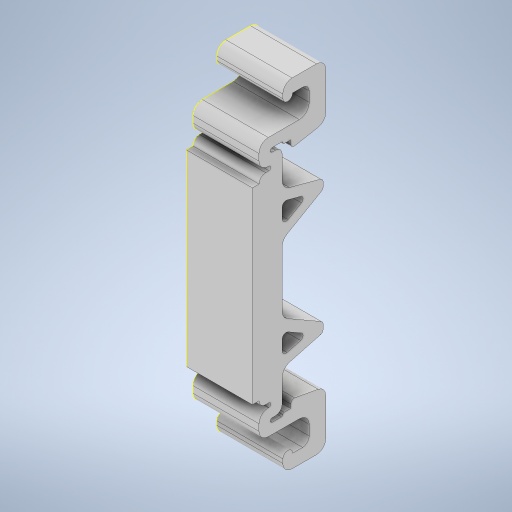
# Autodesk Inventor part: DIN-rail-mount
Saved by Autodesk Inventor 2023 (Build 270158030, 158C)
## iProperties
Created: 2024-03-20
Part Number: DIN-rail-mount
Material: Generic
Document SubType Name: Modeling
Designer: Imogen Heard
Density: 1 g/cm^3
Appearance: Default
Author: Imogen Heard
Autodesk Inventor part; units mm, degrees
ref_plane "YZ Plane" through (0, 0, 0) normal (1, 0, 0) x (0, 1, 0)
ref_plane "XZ Plane" through (0, 0, 0) normal (0, 1, 0) x (-1, 0, 0)
ref_plane "XY Plane" through (0, 0, 0) normal (0, 0, 1) x (1, 0, 0)
sketch "DIN-rail-clip-generic-V1.0" plane through (0, 0, 0) normal (0, 0, 1) x (1, 0, 0)
  line L0 (0, 40.9467) -> (3, 40.9467)
  line L1 (3, 40.9467) -> (3, 17.5)
  line L2 (3, 17.5) -> (0, 17.5)
  line L3 (0, 17.5) -> (0, 40.9467)
  line L4 (0, 35.1) -> (-0.3528, 35.269) construction
  line L5 (-0.3528, 35.269) -> (-1.1784, 35.269) construction
  line L6 (-1.1784, 35.269) -> (-1.277, 34.6657) construction
  line L7 (-1.277, 34.6657) -> (-0.9372, 34.5565) construction
  line L8 (-0.9372, 34.5565) -> (-2.5363, 34.2808) construction
  line L9 (-2.5363, 34.2808) -> (-3.3649, 34.5884) construction
  line L10 (-3.3649, 34.5884) -> (-4.7205, 35.8697) construction
  line L11 (-4.7205, 35.8697) -> (-5.1321, 37.4532) construction
  line L12 (-5.1321, 37.4532) -> (-5.1209, 40.8876) construction
  line L13 (-5.1209, 40.8876) -> (-4.7, 42.1113) construction
  line L14 (-4.7, 42.1113) -> (-3.9, 43.3113) construction
  line L15 (-3.9, 43.3113) -> (-2.1, 44.1113) construction
  line L16 (-2.1, 44.1113) -> (0, 43.5467) construction
  line L17 (0, 43.5467) -> (0.1036, 42.9467) construction
  line L18 (0.1036, 42.9467) -> (-0.2, 41.9467) construction
  line L19 (-0.2, 41.9467) -> (-1.1, 42.4004) construction
  line L20 (-1.1, 42.4004) -> (-2.3, 42.4379) construction
  spline S0 degree 4 poles (0, 35.1) (-0.3528, 35.269) (-1.1784, 35.269) (-1.277, 34.6657) (-0.9372, 34.5565) (-2.5363, 34.2808) (-3.3649, 34.5884) (-4.7205, 35.8697) (-5.1321, 37.4532) (-5.1209, 40.8876) (-4.7, 42.1113) (-3.9, 43.3113) (-2.1, 44.1113) (0, 43.5467) (0.1036, 42.9467) (-0.2, 41.9467) (-1.1, 42.4004) (-2.3, 42.4379) (-2.2829, 41.0379) (-1.7552, 41.1368) (0, 40.9467) knots 1 1 1 1 1 2 3 4 5 6 7 8 9 10 11 12 13 14 15 16 17 17.993985 17.993985 17.993985 17.993985 17.993985
  line L21 (0, 35.8905) -> (-0.7907, 36.0877) construction
  line L22 (-0.7907, 36.0877) -> (-1.1784, 36.0877) construction
  line L23 (-1.1784, 36.0877) -> (-2.2779, 36.5342) construction
  line L24 (-2.2779, 36.5342) -> (-2.7458, 36.6343) construction
  line L25 (-2.7458, 36.6343) -> (-3.471, 38.3527) construction
  line L26 (-3.471, 38.3527) -> (-2.7458, 40.1075) construction
  spline S1 degree 4 poles (0, 35.8905) (-0.7907, 36.0877) (-1.1784, 36.0877) (-2.2779, 36.5342) (-2.7458, 36.6343) (-3.471, 38.3527) (-2.7458, 40.1075) (-2.4429, 40.6075) (-0.7055, 40.4056) (0, 40.2568) knots 1 1 1 1 1 2 3 4 5 6 6.977977 6.977977 6.977977 6.977977 6.977977
  line L27 (-2.3, 42.4379) -> (-2.2829, 41.0379) construction
  line L28 (-2.2829, 41.0379) -> (-1.7552, 41.1368) construction
  line L29 (-1.7552, 41.1368) -> (0, 40.9467) construction
  line L30 (-2.7458, 40.1075) -> (-2.4429, 40.6075) construction
  line L31 (-2.4429, 40.6075) -> (-0.7055, 40.4056) construction
  line L32 (-0.7055, 40.4056) -> (0, 40.2568) construction
  line L33 (0, 36.6343) -> (-1.1784, 36.9758) construction
  line L34 (-1.1784, 36.9758) -> (-2.2101, 37.6402) construction
  line L35 (-2.2101, 37.6402) -> (-2.1452, 38.3006) construction
  line L36 (-2.1452, 38.3006) -> (-1.8076, 39.3817) construction
  line L37 (-1.8076, 39.3817) -> (-0.8778, 39.5886) construction
  line L38 (-0.8778, 39.5886) -> (0, 39.5886) construction
  spline S2 degree 4 poles (0, 36.6343) (-1.1784, 36.9758) (-2.2101, 37.6402) (-2.1452, 38.3006) (-1.8076, 39.3817) (-0.8778, 39.5886) (0, 39.5886) knots 1 1 1 1 1 2 3 4 4 4 4 4
  line L39 (-0.5144, 23.8721) -> (0, 22.0778) construction
  spline S3 degree 4 poles (0, 28.5164) (-0.0002, 28.5161) (-0.1764, 28.1682) (-0.5144, 27.8581) (-1.1668, 26.9412) (-3.3762, 27.1074) (-5.9868, 27.5396) (-6.4206, 26.5054) (-5.8606, 24.9054) (-2.8606, 24.6412) (-1.4606, 24.4656) (-0.5144, 23.8721) (0, 22.0778) knots 1 1 1 1 1 1.050464 1.110527 1.512977 1.739488 1.83789 2 2.236311 2.876473 3 3 3 3 3
  line L40 (-1.4606, 24.4656) -> (-0.5144, 23.8721) construction
  line L41 (-3.3762, 27.1074) -> (-5.9868, 27.5396) construction
  line L42 (-5.9868, 27.5396) -> (-6.4206, 26.5054) construction
  line L43 (-6.4206, 26.5054) -> (-5.8606, 24.9054) construction
  line L44 (-5.8606, 24.9054) -> (-2.8606, 24.6412) construction
  line L45 (-2.8606, 24.6412) -> (-1.4606, 24.4656) construction
  line L46 (0, 28.5164) -> (-0.1764, 28.1682) construction
  line L47 (-0.1764, 28.1682) -> (-0.5144, 27.8581) construction
  line L48 (-0.5144, 27.8581) -> (-1.1668, 26.9412) construction
  line L49 (-1.1668, 26.9412) -> (-3.3762, 27.1074) construction
  circle A0 centre (1, 40.9467) radius 0.7
  point P0 (0, 17.5)
  point P1 (-0.5, 35)
  point P2 (-1, 33.6)
  dimension "d63" = 3
  dimension "d68" = 23.4467
  dimension "d71" = 0.9373
  dimension "d73" = 0.269
  dimension "d74" = 0.3528
  dimension "d79" = 1.5363
  dimension "d85" = 0.7905
  dimension "d87" = 1.1784
  dimension "d88" = 0.7907
  dimension "d89" = 1.5835
  dimension "d90" = 5.1321
  dimension "d92" = 2.2779
  dimension "d93" = 2.7458
  dimension "d95" = 1.7184
  dimension "d96" = 0.7252
  dimension "d97" = 3.4344
  dimension "d99" = 1.2236
  dimension "d100" = 0.4209
  dimension "d101" = 1.2
  dimension "d102" = 0.8
  dimension "d103" = 1.8
  dimension "d104" = 0.8
  dimension "d105" = 2.6
  dimension "d106" = 0.1036
  dimension "d107" = 2
  dimension "d108" = 0.2
  dimension "d109" = 1
  dimension "d110" = 0.9
  dimension "d111" = 0.4536
  dimension "d112" = 1.2
  dimension "d113" = 1.4
  dimension "d114" = 0.0375
  dimension "d115" = 0.0171
  dimension "d116" = 0.5278
  dimension "d117" = 0.0989
  dimension "d118" = 0.69
  dimension "d119" = 0.6682
  dimension "d120" = 0.7055
  dimension "d121" = 0.5412
  dimension "d122" = 1.7374
  dimension "d123" = 0.2019
  dimension "d124" = 0.5
  dimension "d125" = 0.3029
  dimension "d126" = 1.1784
  dimension "d127" = 3.9709
  dimension "d128" = 0.6643
  dimension "d129" = 1.0316
  dimension "d130" = 0.6604
  dimension "d131" = 0.0649
  dimension "d132" = 1.8076
  dimension "d133" = 1.565
  dimension "d134" = 0.9298
  dimension "d136" = 0.7438
  dimension "d138" = 0.3482
  dimension "d139" = 0.3101
  dimension "d140" = 0.9169
  dimension "d141" = 2.2093
  dimension "d142" = 0.1662
  dimension "d143" = 0.1764
  dimension "d144" = 0.3381
  dimension "d145" = 0.6524
  dimension "d147" = 0.4338
  dimension "d148" = 1.6
  dimension "d149" = 0.56
  measures "d63" distance of the line from the sketch origin of L1
  measures "d68" distance between parallel lines of L2 L0
  measures "d73" vertical distance of L4.end point (-0.5, 35)
  measures "d79" horizontal distance of point (-1, 33.6) L8.end
  measures "d85" distance of L21.start L4.start
  measures "d89" vertical distance of L10.end L11.end
  measures "d95" vertical distance of L24.end L25.end
  measures "d96" horizontal distance of L25.end L24.end
  measures "d97" distance of L11.end L12.end
  measures "d99" vertical distance of L12.end L13.end
  measures "d100" horizontal distance of L13.end L12.end
  measures "d101" vertical distance of L14.end L13.end
  measures "d102" horizontal distance of L14.end L13.end
  measures "d103" horizontal distance of L15.end L14.end
  measures "d104" vertical distance of L14.end L15.end
  measures "d105" distance from line of L0 L16.end
  measures "d107" distance from line of L0 L17.end
  measures "d109" distance from line of L0 L18.end
  measures "d110" horizontal distance of L18.end L19.end
  measures "d111" vertical distance of L18.end L19.end
  measures "d112" horizontal distance of L19.end L20.end
  measures "d113" vertical distance of L27.end L20.end
  measures "d114" vertical distance of L20.end L19.end
  measures "d115" horizontal distance of L20.end L27.end
  measures "d116" horizontal distance of L27.end L28.end
  measures "d117" vertical distance of L27.end L28.end
  measures "d118" distance of L29.end L32.end
  measures "d119" distance of L38.end L32.end
  measures "d121" distance from line of L31.end L0
  measures "d122" horizontal distance of L30.end L31.end
  measures "d123" vertical distance of L30.end L31.end
  measures "d124" vertical distance of L26.end L30.end
  measures "d125" horizontal distance of L30.end L26.end
  measures "d127" distance from line of L0 L33.end
  measures "d128" vertical distance of L33.end L34.end
  measures "d129" horizontal distance of L33.end L34.end
  measures "d130" vertical distance of L35.end L34.end
  measures "d131" horizontal distance of L35.end L34.end
  measures "d133" distance from line of L36.end L0
  measures "d134" horizontal distance of L36.end L37.end
  measures "d136" distance of L21.start L33.start
  measures "d138" vertical distance of point (0, 28.516) L46.end
  measures "d139" vertical distance of L46.end L47.end
  measures "d140" vertical distance of L47.end L48.end
  measures "d141" horizontal distance of L49.end L48.end
  measures "d142" vertical distance of L48.end L49.end
  measures "d143" horizontal distance of L46.end point (0, 28.516)
  measures "d144" horizontal distance of L47.end L46.end
  measures "d145" horizontal distance of L47.end L48.end
  measures "d147" horizontal distance of L42.end L41.end
  measures "d148" vertical distance of L42.end L43.end
  measures "d149" horizontal distance of L43.end L42.end
sketch "Sketch1" plane through (0, 0, 0) normal (1, 0, 0) x (0, 1, 0)
  line L0 (5.8, -7.3) -> (29.2, -7.3)
  line L1 (29.2, -6.3) -> (5.8, -6.3)
  line L2 (32.2, -1) -> (35, -1)
  line L3 (35, -1) -> (35, 0)
  line L4 (35, 0) -> (32.2, 0)
  line L5 (-1817770.1114, -20.3632) -> (-1817770.1114, -1)
  line L6 (2.8, 0) -> (0, 0)
  line L7 (0, 0) -> (0, -1)
  line L8 (0, -1) -> (2.8, -1)
  line L9 (4.8, -2) -> (4.8, -5.3)
  arc A0 (32.2, -1) -> (31.2, -2) centre (32.2, -2) ccw
  arc A1 (29.2, -6.3) -> (30.2, -5.3) centre (29.2, -5.3) ccw
  arc A2 (4.8, -5.3) -> (5.8, -6.3) centre (5.8, -5.3) ccw
  arc A3 (3.8, -2) -> (2.8, -1) centre (2.8, -2) ccw
  arc A4 (4.8, -2) -> (2.8, 0) centre (2.8, -2) ccw
  arc A5 (3.8, -5.3) -> (5.8, -7.3) centre (5.8, -5.3) ccw
  line L10 (3.8, -2) -> (3.8, -5.3)
  arc A6 (32.2, 0) -> (30.2, -2) centre (32.2, -2) ccw
  arc A7 (29.2, -7.3) -> (31.2, -5.3) centre (29.2, -5.3) ccw
  line L11 (31.2, -2) -> (31.2, -5.3)
  line L12 (30.2, -2) -> (30.2, -5.3)
  line L13 (17.5, -4.8951) -> (17.5, -40.6352) construction
  point P0 (4.8, -3.65)
  dimension "d0" = 1
  dimension "d1" = 1
  dimension "d5" = 35
  dimension "d8" = 7.3
  dimension "d9" = 1
  dimension "d10" = 1
  dimension "d11" = 2
  dimension "d12" = 2
  dimension "d13" = 12.7
  dimension "d15" = 12.7
  dimension "d16" = 4.8
  dimension "d17" = 4.8
  dimension "d20" = 1
  dimension "d21" = 1
  dimension "d22" = 2
  constraints: 28 end point, 17 point on circle, 12 tangent, 8 centre point, 7 horizontal alignment, 4 equal radius, 4 parallel, 3 perpendicular, 2 horizontal, 2 vertical, 1 coincident, 1 midpoint, 1 point on line, 1 vertical alignment
  measures "d0" distance between parallel lines of L2 L4
  measures "d1" distance between parallel lines of L0 L1
  measures "d5" distance between parallel lines of L7 L3
  measures "d8" distance between parallel lines of L4 L0
  measures "d9" radius of A0
  measures "d10" radius of A1
  measures "d11" radius of A4
  measures "d12" radius of A6
  measures "d13" distance between parallel lines of L13 L12
  measures "d15" distance between parallel lines of L13 L9
  measures "d16" distance between parallel lines of L9 L7
  measures "d17" distance between parallel lines of L12 L3
  measures "d20" distance between parallel lines of L12 L11
  measures "d21" distance between parallel lines of L10 L9
  measures "d22" radius of A5
extrude "Extrusion5" add sketch "Sketch1" along normal blind 10
sketch "Sketch6" plane through (0, 0, 0) normal (1, 0, 0) x (0, 1, 0)
  arc A0 (3.8, -5.3) -> (5.8, -7.3) centre (5.8, -5.3) ccw projected
  line L0 (5.8, -7.3) -> (29.2, -7.3) projected
  arc A1 (29.2, -7.3) -> (31.2, -5.3) centre (29.2, -5.3) ccw projected
  line L1 (31.2, -5.3) -> (31.2, -2) projected
  line L2 (32.2, -1) -> (35, -1) projected
  arc A2 (32.2, 0) -> (30.2, -2) centre (32.2, -2) ccw projected
  line L3 (30.2, -2) -> (30.2, -5.3) projected
  line L4 (29.2, -6.3) -> (5.8, -6.3) projected
  line L5 (4.8, -5.3) -> (4.8, -2) projected
  arc A3 (4.8, -2) -> (2.8, 0) centre (2.8, -2) ccw projected
  line L6 (2.8, 0) -> (0, 0) projected
  line L7 (0, 0) -> (0, -1) projected
  line L8 (0, -1) -> (2.8, -1) projected
  line L9 (3.8, -2) -> (3.8, -5.3) projected
  line L10 (37.1, 0.1) -> (37.1, -2.5)
  line L11 (37.1, -6.5) -> (36.0383, -6.5)
  line L12 (35.1, -6.139) -> (35.1, -0.2)
  line L13 (38.6, -4) -> (40.1, -4)
  line L14 (43.1, -4) -> (43.1, -5.1)
  line L15 (41.7, -6.5) -> (37.1, -6.5)
  line L16 (37.1, -6.5) -> (37.1, -4)
  line L17 (43.1, -4) -> (41.3737, -4)
  line L18 (35.1, -1.2) -> (34.5, -1.2)
  line L19 (34.0082, -1.7902) -> (34.6613, -5.3525)
  line L20 (43.1, -4) -> (41.1, -4)
  line L21 (41.1, -3) -> (41.1, 0)
  line L22 (41.1, 0) -> (41.7, 0)
  line L23 (43.1, -1.4) -> (43.1, -4)
  line L24 (21.7381, 0.1) -> (17.5, 0.1)
  line L25 (17.5, 0.1) -> (17.5, 3.6)
  line L26 (34.7, 3.6) -> (35.7, 3.6)
  line L27 (37.1, 2.2) -> (37.1, 0.1)
  line L28 (32.7, 2.6) -> (32.7, 2.1)
  line L29 (32.7, 2.1) -> (32.7, 2.6809)
  line L30 (33.3, 2.1) -> (33.3, 2.2)
  arc A4 (37.1, 2.2) -> (35.7, 3.6) centre (35.7, 2.2) ccw
  arc A5 (34.6613, -5.3525) -> (36.0383, -6.5) centre (36.0383, -5.1) ccw
  arc A6 (41.7, -6.5) -> (43.1, -5.1) centre (41.7, -5.1) ccw
  arc A7 (43.1, -1.4) -> (41.7, 0) centre (41.7, -1.4) ccw
  arc A8 (37.1, -2.5) -> (38.6, -4) centre (38.6, -2.5) ccw
  arc A9 (34.7, 3.6) -> (33.3, 2.2) centre (34.7, 2.2) ccw
  arc A10 (32.7, 2.1) -> (33.3, 2.1) centre (33, 2.1) ccw
  line L31 (31.7, 3.6) -> (17.5, 3.6)
  line L32 (17.5, 3.6) -> (17.5, 0.1)
  line L33 (30.3959, 0.1) -> (32.7, 0.1)
  line L34 (32.7, 0.1) -> (32.7, 2.6)
  circle A11 centre (41.1, -0.75) radius 0.75
  arc A12 (34.5, -1.2) -> (34.0082, -1.7902) centre (34.5, -1.7) ccw
  arc A13 (40.1, -4) -> (41.1, -3) centre (40.1, -3) ccw
  line L35 (17.5, 3.6) -> (31.7, 3.6)
  line L36 (31.7, 3.6) -> (31.7, 4.6)
  line L37 (31.7, 4.6) -> (17.5, 4.6)
  line L38 (17.5, 4.6) -> (17.5, 3.6)
  line L39 (28.9471, -1.0118) -> (27.683, -5.7294)
  line L40 (29.2, -6.3) -> (5.8, -6.3) projected
  line L41 (26.0393, -5.85) -> (23.0371, -0.65)
  line L42 (27.2, -6.1) -> (26.4723, -6.1)
  line L43 (27.4897, -0.6553) -> (26.9407, -2.7041)
  line L44 (26.0247, -2.8247) -> (24.8558, -0.8)
  arc A14 (30.3959, 0.1) -> (28.9471, -1.0118) centre (30.3959, -1.4) ccw
  arc A15 (23.0371, -0.65) -> (21.7381, 0.1) centre (21.7381, -1.4) ccw
  arc A16 (26.0247, -2.8247) -> (26.9407, -2.7041) centre (26.4577, -2.5747) ccw
  arc A17 (27.2, -6.1) -> (27.683, -5.7294) centre (27.2, -5.6) ccw
  arc A18 (26.0393, -5.85) -> (26.4723, -6.1) centre (26.4723, -5.6) ccw
  line L45 (26.9101, 0.1) -> (25.3754, 0.1)
  arc A19 (27.4897, -0.6553) -> (26.9101, 0.1) centre (26.9101, -0.5) ccw
  arc A20 (25.3754, 0.1) -> (24.8558, -0.8) centre (25.3754, -0.5) ccw
  line L46 (35, -1) -> (35, 0) projected
  line L47 (35.5, 0.2) -> (35.5, 1.6)
  line L48 (34.9, 1.6) -> (34.9, 1.1)
  arc A21 (35.5, 1.6) -> (35.2, 1.9) centre (35.2, 1.6) ccw
  arc A22 (35.2, 1.9) -> (34.9, 1.6) centre (35.2, 1.6) ccw
  line L49 (32.7, 0.1) -> (33.9, 0.1)
  arc A23 (33.9, 0.1) -> (34.9, 1.1) centre (33.9, 1.1) ccw
  arc A24 (32.7, 2.6) -> (31.7, 3.6) centre (31.7, 2.6) ccw
  arc A25 (3.8, -5.3) -> (5.8, -7.3) centre (5.8, -5.3) ccw projected
  line L50 (3.8, -2) -> (3.8, -5.3) projected
  arc A26 (3.8, -2) -> (2.8, -1) centre (2.8, -2) ccw projected
  line L51 (0, -1) -> (2.8, -1) projected
  line L52 (0, 0) -> (0, -1) projected
  line L53 (2.8, 0) -> (0, 0) projected
  arc A27 (4.8, -2) -> (2.8, 0) centre (2.8, -2) ccw projected
  line L54 (4.8, -5.3) -> (4.8, -2) projected
  arc A28 (4.8, -5.3) -> (5.8, -6.3) centre (5.8, -5.3) ccw projected
  line L55 (29.2, -6.3) -> (5.8, -6.3) projected
  arc A29 (29.2, -6.3) -> (30.2, -5.3) centre (29.2, -5.3) ccw projected
  line L56 (30.2, -2) -> (30.2, -5.3) projected
  arc A30 (32.2, 0) -> (30.2, -2) centre (32.2, -2) ccw projected
  line L57 (35, 0) -> (32.2, 0) projected
  line L58 (35, -1) -> (35, 0) projected
  line L59 (32.2, -1) -> (35, -1) projected
  arc A31 (32.2, -1) -> (31.2, -2) centre (32.2, -2) ccw projected
  line L60 (31.2, -5.3) -> (31.2, -2) projected
  arc A32 (29.2, -7.3) -> (31.2, -5.3) centre (29.2, -5.3) ccw projected
  line L61 (5.8, -7.3) -> (29.2, -7.3) projected
  line L62 (35.3, 0) -> (35.3, 0)
  line L63 (35, 0) -> (32.2, 0) projected
  arc A33 (35.3, 0) -> (35.5, 0.2) centre (35.3, 0.2) ccw
  arc A34 (35.3, 0) -> (35.1, -0.2) centre (35.3, -0.2) ccw
  point P0 (43.1, -6.5)
  point P1 (33.9, -1.2)
  point P2 (17.5, -6.3)
  point P3 (41.1, 0)
  point P4 (41.1, -1.5)
  point P5 (32.922, 3.2)
  point P6 (27.5837, -6.1)
  point P7 (26.1837, -6.1)
  point P8 (22.6041, 0.1)
  point P9 (27.692, 0.1)
  point P10 (24.3361, 0.1)
  point P11 (35.1, -5.9421)
  point P12 (41.1, 0)
  point P13 (34.8, -1.2)
  point P14 (37.1, 1.15)
  point P15 (35.2, 3.6)
  point P16 (35.1, 0)
  point P17 (35.5, 0)
  point P18 (35.2, 1.9)
  point P19 (17.5, 3.7)
  point P20 (32.8, 3.3)
  point P21 (33.3, 1.7)
  point P22 (35.1, 0)
  point P23 (35.3, 3.7)
  point P24 (34.9, 1.35)
  point P25 (35.3, 0)
  dimension "d259" = 2.5
  dimension "d268" = 6
  dimension "d269" = 2
  dimension "d270" = 4
  dimension "d279" = 3
  dimension "d283" = 1.5
  dimension "d290" = 1.5
  dimension "d291" = 0.75
  dimension "d293" = 1
  dimension "d295" = 1
  dimension "d298" = 75
  dimension "d299" = 60
  dimension "d300" = 0.2
  dimension "d301" = 1.4
  dimension "d303" = 1.5
  dimension "d304" = 1.5
  dimension "d305" = 1.5
  dimension "d306" = 1.5
  dimension "d307" = 0.5
  dimension "d320" = 0.2
  dimension "d322" = 0.1
  dimension "d333" = 0.1
  dimension "d334" = 0.2
  dimension "d338" = 2
  dimension "d339" = 3
  dimension "d340" = 0.6
  dimension "d341" = 0.6
  dimension "d342" = 1.6
  dimension "d343" = 1.6
  dimension "d344" = 1.4
  dimension "d345" = 1.4
  dimension "d346" = 0.3
  dimension "d348" = 3.5
  dimension "d349" = 2
  dimension "d350" = 1
  dimension "d351" = 0.3
  dimension "d354" = 0.2
  dimension "d355" = 0.6
  dimension "d356" = 1.2
  dimension "d357" = 0.5
  dimension "d358" = 1.4
  dimension "d359" = 1.4
  dimension "d360" = 0.6
  dimension "d361" = 2
  constraints: 78 end point, 45 point on circle, 42 tangent, 32 point on line, 27 centre point, 14 parallel, 8 horizontal, 7 equal radius, 5 midpoint, 5 perpendicular, 4 horizontal alignment, 4 vertical alignment, 2 coincident, 1 collinear, 5 other
  measures "d259" distance between parallel lines of L15 L13
  measures "d268" distance between parallel lines of L10 L14
  measures "d269" distance between parallel lines of L21 L23
  measures "d270" distance between parallel lines of L22 L13
  measures "d279" distance between parallel lines of L13 L2
  measures "d283" radius of A8
  measures "d290" diameter of A11
  measures "d291" distance from line of L22 A11.centre
  measures "d293" radius of A13
  measures "d295" distance between parallel lines of L35 L37
  measures "d298" angle of L24 L39
  measures "d299" angle of L24 L41
  measures "d300" distance from line of L4 point (26.184, -6.1)
  measures "d301" distance of point (27.584, -6.1) point (26.184, -6.1)
  measures "d303" distance between parallel lines of L41 L44
  measures "d304" distance between parallel lines of L39 L43
  measures "d305" radius of A14
  measures "d306" radius of A15
  measures "d307" radius of A16
  measures "d320" distance from line of point (34.8, -1.2) L2
  measures "d322" distance between parallel lines of L46 L12
  measures "d333" distance between parallel lines of L57 L49
  measures "d334" radius of A33
  measures "d338" distance from line of A10.centre L49
  measures "d339" distance from line of L3 A17.centre
  measures "d340" radius of A19
  measures "d341" distance from line of point (34.9, 1.35) L47
  measures "d342" distance between parallel lines of L48 L30
  measures "d343" distance between parallel lines of L27 L47
  measures "d344" radius of A4
  measures "d345" radius of A9
  measures "d346" radius of A21
  measures "d348" distance between parallel lines of L33 L31
  measures "d349" distance between parallel lines of L10 L12
  measures "d350" radius of A23
  measures "d351" radius of A10
  measures "d354" radius of A34
  measures "d355" distance between parallel lines of L28 L30
  measures "d356" distance from line of L12 point (33.9, -1.2)
  measures "d357" radius of A12
  measures "d358" radius of A7
  measures "d359" radius of A5
  measures "d360" distance from line of L12 A12.centre
  measures "d361" distance from line of L26 A21.centre
extrude "Extrusion6" add sketch "Sketch6" along normal blind 10 separate body contours L10 A8 L13 A13 L21 A11 L22 A7 L23 L14 A6 L15 L11 A5 L12 A34 A33 L47 A21 A22 L48 A23 L49 L34 A10 L30 A9 L26 A4 L27 | A11 L21 | L21 A11 | L34 L33 A14 L39 A17 L42 A18 L41 A15 L24 L25 L31 A24 L28 | L31 L38 L37 L36 | A5 L19 A12 L18 L12
mirror "Mirror2" about plane through (0, 17.5, 4.6) normal (0, -1, 0) of "Extrusion6"
sketch "Sketch7" plane through (0, 0, 0) normal (-1, 0, 0) x (0, 0, 1)
  arc A0 (-0.6553, 7.5103) -> (0.1, 8.0899) centre (-0.5, 8.0899) ccw projected
  line L0 (-0.6553, 7.5103) -> (-2.7041, 8.0593) projected
  arc A1 (-2.8247, 8.9753) -> (-2.7041, 8.0593) centre (-2.5747, 8.5423) ccw projected
  line L1 (-2.8247, 8.9753) -> (-0.8, 10.1442) projected
  arc A2 (0.1, 9.6246) -> (-0.8, 10.1442) centre (-0.5, 9.6246) ccw projected
  line L2 (0.1, 9.6246) -> (0.1, 8.0899) projected
  line L3 (0.1, 30.3959) -> (0.1, 33.9) projected
  arc A3 (-1.0118, 28.9471) -> (0.1, 30.3959) centre (-1.4, 30.3959) ccw projected
  line L4 (-5.7294, 27.683) -> (-1.0118, 28.9471) projected
  arc A4 (-5.7294, 27.683) -> (-6.1, 27.2) centre (-5.6, 27.2) ccw projected
  line L5 (-6.1, 26.4723) -> (-6.1, 27.2) projected
  arc A5 (-6.1, 26.4723) -> (-5.85, 26.0393) centre (-5.6, 26.4723) ccw projected
  line L6 (-0.65, 23.0371) -> (-5.85, 26.0393) projected
  arc A6 (0.1, 21.7381) -> (-0.65, 23.0371) centre (-1.4, 21.7381) ccw projected
  line L7 (0.1, 21.7381) -> (0.1, 13.2619) projected
  arc A7 (-0.65, 11.9629) -> (0.1, 13.2619) centre (-1.4, 13.2619) ccw projected
  line L8 (-0.65, 11.9629) -> (-5.85, 8.9607) projected
  arc A8 (-5.85, 8.9607) -> (-6.1, 8.5277) centre (-5.6, 8.5277) ccw projected
  line L9 (-6.1, 8.5277) -> (-6.1, 7.8) projected
  arc A9 (-6.1, 7.8) -> (-5.7294, 7.317) centre (-5.6, 7.8) ccw projected
  line L10 (-5.7294, 7.317) -> (-1.0118, 6.0529) projected
  arc A10 (0.1, 4.6041) -> (-1.0118, 6.0529) centre (-1.4, 4.6041) ccw projected
  line L11 (0.1, 4.6041) -> (0.1, 1.1) projected
  arc A11 (0.1, 1.1) -> (1.1, 0.1) centre (1.1, 1.1) ccw projected
  line L12 (1.1, 0.1) -> (1.6, 0.1) projected
  arc A12 (1.6, -0.5) -> (1.6, 0.1) centre (1.6, -0.2) ccw projected
  line L13 (1.6, -0.5) -> (0.2, -0.5) projected
  arc A13 (0, -0.3) -> (0.2, -0.5) centre (0.2, -0.3) ccw projected
  arc A14 (0, -0.3) -> (-0.2, -0.1) centre (-0.2, -0.3) ccw projected
  line L14 (-0.2, -0.1) -> (-1.2, -0.1) projected
  line L15 (-1.2, -0.1) -> (-1.2, 0.5) projected
  arc A15 (-1.2, 0.5) -> (-1.7902, 0.9918) centre (-1.7, 0.5) ccw projected
  line L16 (-1.7902, 0.9918) -> (-5.3525, 0.3387) projected
  arc A16 (-5.3525, 0.3387) -> (-6.5, -1.0383) centre (-5.1, -1.0383) ccw projected
  line L17 (-6.5, -1.0383) -> (-6.5, -6.7) projected
  arc A17 (-6.5, -6.7) -> (-5.1, -8.1) centre (-5.1, -6.7) ccw projected
  line L18 (-5.1, -8.1) -> (-1.4, -8.1) projected
  arc A18 (-1.4, -8.1) -> (0, -6.7) centre (-1.4, -6.7) ccw projected
  line L19 (0, -6.7) -> (0, -6.1) projected
  arc A19 (0, -6.1) -> (-1.5, -6.1) centre (-0.75, -6.1) ccw projected
  line L20 (-1.5, -6.1) -> (-3, -6.1) projected
  arc A20 (-4, -5.1) -> (-3, -6.1) centre (-3, -5.1) ccw projected
  line L21 (-4, -5.1) -> (-4, -3.6) projected
  arc A21 (-2.5, -2.1) -> (-4, -3.6) centre (-2.5, -3.6) ccw projected
  line L22 (-2.5, -2.1) -> (2.2, -2.1) projected
  arc A22 (2.2, -2.1) -> (3.6, -0.7) centre (2.2, -0.7) ccw projected
  line L23 (3.6, -0.7) -> (3.6, 0.3) projected
  arc A23 (3.6, 0.3) -> (2.2, 1.7) centre (2.2, 0.3) ccw projected
  line L24 (2.2, 1.7) -> (2.1, 1.7) projected
  arc A24 (2.1, 2.3) -> (2.1, 1.7) centre (2.1, 2) ccw projected
  line L25 (2.1, 2.3) -> (2.6, 2.3) projected
  arc A25 (2.6, 2.3) -> (3.6, 3.3) centre (2.6, 3.3) ccw projected
  line L26 (3.6, 3.3) -> (4.6, 3.3) projected
  line L27 (4.6, 31.7) -> (4.6, 3.3) projected
  line L28 (3.6, 31.7) -> (4.6, 31.7) projected
  arc A26 (3.6, 31.7) -> (2.6, 32.7) centre (2.6, 31.7) ccw projected
  line L29 (2.1, 32.7) -> (2.6, 32.7) projected
  arc A27 (2.1, 33.3) -> (2.1, 32.7) centre (2.1, 33) ccw projected
  line L30 (2.2, 33.3) -> (2.1, 33.3) projected
  arc A28 (2.2, 33.3) -> (3.6, 34.7) centre (2.2, 34.7) ccw projected
  line L31 (3.6, 35.7) -> (3.6, 34.7) projected
  arc A29 (3.6, 35.7) -> (2.2, 37.1) centre (2.2, 35.7) ccw projected
  line L32 (-2.5, 37.1) -> (2.2, 37.1) projected
  arc A30 (-4, 38.6) -> (-2.5, 37.1) centre (-2.5, 38.6) ccw projected
  line L33 (-4, 40.1) -> (-4, 38.6) projected
  arc A31 (-3, 41.1) -> (-4, 40.1) centre (-3, 40.1) ccw projected
  line L34 (-1.5, 41.1) -> (-3, 41.1) projected
  arc A32 (-1.5, 41.1) -> (0, 41.1) centre (-0.75, 41.1) ccw projected
  line L35 (0, 41.7) -> (0, 41.1) projected
  arc A33 (0, 41.7) -> (-1.4, 43.1) centre (-1.4, 41.7) ccw projected
  line L36 (-5.1, 43.1) -> (-1.4, 43.1) projected
  arc A34 (-5.1, 43.1) -> (-6.5, 41.7) centre (-5.1, 41.7) ccw projected
  line L37 (-6.5, 36.0383) -> (-6.5, 41.7) projected
  arc A35 (-6.5, 36.0383) -> (-5.3525, 34.6613) centre (-5.1, 36.0383) ccw projected
  line L38 (-1.7902, 34.0082) -> (-5.3525, 34.6613) projected
  arc A36 (-1.7902, 34.0082) -> (-1.2, 34.5) centre (-1.7, 34.5) ccw projected
  line L39 (-1.2, 35.1) -> (-1.2, 34.5) projected
  line L40 (-0.2, 35.1) -> (-1.2, 35.1) projected
  arc A37 (-0.2, 35.1) -> (0, 35.3) centre (-0.2, 35.3) ccw projected
  arc A38 (0.2, 35.5) -> (0, 35.3) centre (0.2, 35.3) ccw projected
  line L41 (1.6, 35.5) -> (0.2, 35.5) projected
  arc A39 (1.6, 34.9) -> (1.6, 35.5) centre (1.6, 35.2) ccw projected
  line L42 (1.1, 34.9) -> (1.6, 34.9) projected
  arc A40 (1.1, 34.9) -> (0.1, 33.9) centre (1.1, 33.9) ccw projected
  arc A41 (0.1, 26.9101) -> (-0.6553, 27.4897) centre (-0.5, 26.9101) ccw projected
  line L43 (0.1, 25.3754) -> (0.1, 26.9101) projected
  arc A42 (-0.8, 24.8558) -> (0.1, 25.3754) centre (-0.5, 25.3754) ccw projected
  line L44 (-2.8247, 26.0247) -> (-0.8, 24.8558) projected
  arc A43 (-2.7041, 26.9407) -> (-2.8247, 26.0247) centre (-2.5747, 26.4577) ccw projected
  line L45 (-0.6553, 27.4897) -> (-2.7041, 26.9407) projected
  point P0 (0, 0)
